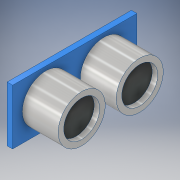
# Autodesk Inventor part: Sonar
Saved by Autodesk Inventor 2018 (Build 220112000, 112)
## iProperties
Created: 2018-02-19
Part Number: Sonar
Material: Generic
Document SubType Name: Modeling
Designer: Melda
Density: 1 g/cm^3
Appearance: Cyan
Author: Melda
Autodesk Inventor part; units mm, degrees
ref_plane "YZ Plane" through (0, 0, 0) normal (1, 0, 0) x (0, 1, 0)
ref_plane "XZ Plane" through (0, 0, 0) normal (0, 1, 0) x (-1, 0, 0)
ref_plane "XY Plane" through (0, 0, 0) normal (0, 0, 1) x (1, 0, 0)
sketch "Sketch1" plane through (0, 0, 0) normal (1, 0, 0) x (0, 1, 0)
  line L0 (11.9118, 21.1765) -> (-8.0882, 21.1765)
  line L1 (-8.0882, 21.1765) -> (-8.0882, -23.8235)
  line L2 (-8.0882, -23.8235) -> (11.9118, -23.8235)
  line L3 (11.9118, -23.8235) -> (11.9118, 21.1765)
  point P0 (0, 0)
  dimension "d0" = 45
  dimension "d1" = 20
  constraints: 8 end point, 2 parallel, 1 horizontal, 1 perpendicular
  measures "d0" distance of L2.end L0.start
  measures "d1" distance of L0.start L0.end
extrude "Extrusion1" add sketch "Sketch1" along normal blind 2
sketch "Sketch2" plane through (2, 0, 0) normal (1, 0, 0) x (0, 0, -1)
  circle A0 centre (-9.1765, 1.9118) radius 8.5
  circle A1 centre (11.8235, 1.9118) radius 8.5
  line L0 (23.8235, 11.9118) -> (-21.1765, 11.9118) projected
  line L1 (-21.1765, 11.9118) -> (-21.1765, -8.0882) projected
  line L2 (23.8235, -8.0882) -> (23.8235, 11.9118) projected
  point P0 (0, 0)
  dimension "d4" = 17
  dimension "d5" = 10
  dimension "d6" = 10
  dimension "d7" = 12
  dimension "d8" = 12
  constraints: 2 centre point, 1 equal radius
  measures "d4" diameter of A0
  measures "d5" distance from line of L0 A0.centre
  measures "d6" distance from line of L0 A1.centre
  measures "d7" distance from line of L1 A0.centre
  measures "d8" distance from line of L2 A1.centre
extrude "Extrusion2" add sketch "Sketch2" along normal blind 13
sketch "Sketch3" plane through (15, 1.9118, 9.1765) normal (1, 0, 0) x (0, 0, -1)
  circle A0 centre (0, 0) radius 6.5
  circle A1 centre (21, 0) radius 6.5
  circle A2 centre (21, 0) radius 8.5 projected
  circle A3 centre (0, 0) radius 8.5 projected
  point P0 (9.1765, -1.9118)
  dimension "d11" = 13
  constraints: 2 centre point, 2 concentric, 1 equal radius
  measures "d11" diameter of A0
extrude "Extrusion3" cut sketch "Sketch3" against normal blind 2 contours A0 | A1
equation "\"d6\" = d5"
equation "\"d8\" = d7"
body "Solid1"
